Autodesk Fusion 360 part; units mm, degrees
(part 3 of 3)
  spline S37 degree 5 poles (17.7781, 0.5617) (17.7707, 0.5659) (17.756, 0.5742) (17.7338, 0.5867) (17.7042, 0.6032) (17.6672, 0.6236) (17.6301, 0.6437) (17.593, 0.6637) (17.5559, 0.6835) (17.5187, 0.7031) (17.4815, 0.7225) (17.4443, 0.7416) (17.407, 0.7606) (17.3696, 0.7793) (17.3323, 0.7978) (17.2949, 0.8161) (17.2574, 0.8342) (17.22, 0.8521) (17.1824, 0.8698) (17.1449, 0.8872) (17.1073, 0.9045) (17.0697, 0.9215) (17.0321, 0.9382) (16.9944, 0.9548) (16.9567, 0.9711) (16.919, 0.9872) (16.8813, 1.0031) (16.8435, 1.0187) (16.8057, 1.0341) (16.7678, 1.0493) (16.73, 1.0642) (16.6921, 1.0789) (16.6542, 1.0933) (16.6163, 1.1075) (16.5783, 1.1214) (16.5403, 1.1351) (16.5023, 1.1486) (16.4643, 1.1618) (16.4263, 1.1747) (16.3882, 1.1874) (16.3501, 1.1998) (16.312, 1.2119) (16.2739, 1.2238) (16.2358, 1.2354) (16.1976, 1.2467) (16.1595, 1.2577) (16.1213, 1.2684) (16.0831, 1.2789) (16.0449, 1.2891) (16.0067, 1.2989) (15.9685, 1.3085) (15.9303, 1.3177) (15.892, 1.3266) (15.8538, 1.3352) (15.8155, 1.3434) (15.7773, 1.3513) (15.7391, 1.3589) (15.7008, 1.3662) (15.6625, 1.3731) (15.6243, 1.3797) (15.5861, 1.3859) (15.5478, 1.3915) (15.5096, 1.3966) (15.4714, 1.4011) (15.4332, 1.4052) (15.395, 1.4089) (15.3568, 1.4124) (15.3186, 1.4156) (15.2805, 1.4184) (15.2424, 1.4204) (15.2044, 1.4214) (15.174, 1.4209) (15.1513, 1.4197) (15.1361, 1.4185) (15.1285, 1.4178) knots -1 -1 -1 -1 -1 -1 -0.98571429 -0.97142857 -0.95714286 -0.94285714 -0.92857143 -0.91428571 -0.9 -0.88571429 -0.87142857 -0.85714286 -0.84285714 -0.82857143 -0.81428571 -0.8 -0.78571429 -0.77142857 -0.75714286 -0.74285714 -0.72857143 -0.71428571 -0.7 -0.68571429 -0.67142857 -0.65714286 -0.64285714 -0.62857143 -0.61428571 -0.6 -0.58571429 -0.57142857 -0.55714286 -0.54285714 -0.52857143 -0.51428571 -0.5 -0.48571429 -0.47142857 -0.45714286 -0.44285714 -0.42857143 -0.41428571 -0.4 -0.38571429 -0.37142857 -0.35714286 -0.34285714 -0.32857143 -0.31428571 -0.3 -0.28571429 -0.27142857 -0.25714286 -0.24285714 -0.22857143 -0.21428571 -0.2 -0.18571429 -0.17142857 -0.15714286 -0.14285714 -0.12857143 -0.11428571 -0.1 -0.08571429 -0.07142857 -0.05714286 -0.04285714 -0.02857143 -0.01428571 0 0 0 0 0 0
  line L37 (15.1285, 1.4178) -> (14.5093, 1.3603)
  arc A75 (14.0753, 1.7104) -> (14.5093, 1.3603) centre (14.4723, 1.7586) ccw
  arc A76 (14.0753, 1.7104) -> (13.9149, 2.7228) centre (0, 0) ccw
  arc A77 (14.2195, 3.1899) -> (13.9149, 2.7228) centre (14.3075, 2.7996) ccw
  line L38 (14.2195, 3.1899) -> (14.8262, 3.3266)
  spline S38 degree 5 poles (14.8262, 3.3266) (14.8336, 3.3282) (14.8484, 3.3318) (14.8704, 3.3376) (14.8995, 3.3466) (14.9353, 3.3592) (14.9709, 3.373) (15.0063, 3.3874) (15.0416, 3.4023) (15.0769, 3.4173) (15.112, 3.4327) (15.1471, 3.4484) (15.1821, 3.4645) (15.2168, 3.4811) (15.2515, 3.4983) (15.2859, 3.516) (15.3203, 3.5341) (15.3545, 3.5525) (15.3886, 3.5713) (15.4227, 3.5903) (15.4566, 3.6096) (15.4904, 3.6293) (15.5242, 3.6492) (15.5578, 3.6695) (15.5913, 3.6901) (15.6247, 3.711) (15.658, 3.7322) (15.6911, 3.7537) (15.7242, 3.7754) (15.7572, 3.7974) (15.7901, 3.8197) (15.8229, 3.8422) (15.8556, 3.865) (15.8882, 3.8881) (15.9206, 3.9114) (15.953, 3.935) (15.9853, 3.9588) (16.0175, 3.9828) (16.0496, 4.0071) (16.0816, 4.0317) (16.1134, 4.0564) (16.1452, 4.0814) (16.1769, 4.1066) (16.2085, 4.1321) (16.24, 4.1577) (16.2714, 4.1836) (16.3027, 4.2098) (16.3339, 4.2361) (16.365, 4.2626) (16.396, 4.2894) (16.4269, 4.3163) (16.4577, 4.3435) (16.4884, 4.3709) (16.519, 4.3985) (16.5495, 4.4263) (16.5799, 4.4543) (16.6103, 4.4825) (16.6405, 4.5108) (16.6706, 4.5394) (16.7006, 4.5682) (16.7305, 4.5972) (16.7603, 4.6263) (16.79, 4.6557) (16.8196, 4.6853) (16.8492, 4.715) (16.8786, 4.7449) (16.9079, 4.775) (16.9371, 4.8053) (16.9662, 4.8358) (16.9952, 4.8664) (17.0241, 4.8973) (17.0471, 4.9221) (17.0644, 4.9408) (17.0759, 4.9533) (17.0816, 4.9595) knots 0 0 0 0 0 0 0.01428571 0.02857143 0.04285714 0.05714286 0.07142857 0.08571429 0.1 0.11428571 0.12857143 0.14285714 0.15714286 0.17142857 0.18571429 0.2 0.21428571 0.22857143 0.24285714 0.25714286 0.27142857 0.28571429 0.3 0.31428571 0.32857143 0.34285714 0.35714286 0.37142857 0.38571429 0.4 0.41428571 0.42857143 0.44285714 0.45714286 0.47142857 0.48571429 0.5 0.51428571 0.52857143 0.54285714 0.55714286 0.57142857 0.58571429 0.6 0.61428571 0.62857143 0.64285714 0.65714286 0.67142857 0.68571429 0.7 0.71428571 0.72857143 0.74285714 0.75714286 0.77142857 0.78571429 0.8 0.81428571 0.82857143 0.84285714 0.85714286 0.87142857 0.88571429 0.9 0.91428571 0.92857143 0.94285714 0.95714286 0.97142857 0.98571429 1 1 1 1 1 1
  arc A78 (17.0816, 4.9595) -> (16.7344, 6.028) centre (0, 0) ccw
  spline S39 degree 5 poles (16.7344, 6.028) (16.7261, 6.0297) (16.7095, 6.033) (16.6846, 6.038) (16.6513, 6.0445) (16.6098, 6.0525) (16.5683, 6.0602) (16.5269, 6.0678) (16.4854, 6.0751) (16.444, 6.0823) (16.4027, 6.0892) (16.3613, 6.0959) (16.32, 6.1024) (16.2787, 6.1087) (16.2374, 6.1147) (16.1962, 6.1206) (16.155, 6.1262) (16.1138, 6.1317) (16.0727, 6.1369) (16.0316, 6.1419) (15.9906, 6.1466) (15.9495, 6.1512) (15.9086, 6.1555) (15.8676, 6.1596) (15.8267, 6.1635) (15.7859, 6.1672) (15.7451, 6.1706) (15.7043, 6.1738) (15.6636, 6.1767) (15.6229, 6.1795) (15.5823, 6.182) (15.5417, 6.1842) (15.5012, 6.1862) (15.4608, 6.188) (15.4204, 6.1895) (15.38, 6.1908) (15.3397, 6.1919) (15.2995, 6.1927) (15.2593, 6.1932) (15.2192, 6.1935) (15.1791, 6.1935) (15.1392, 6.1933) (15.0992, 6.1928) (15.0594, 6.192) (15.0196, 6.191) (14.9799, 6.1897) (14.9403, 6.1881) (14.9008, 6.1862) (14.8613, 6.1841) (14.8219, 6.1817) (14.7826, 6.179) (14.7434, 6.176) (14.7043, 6.1726) (14.6653, 6.1689) (14.6264, 6.1649) (14.5875, 6.1606) (14.5488, 6.156) (14.5102, 6.1511) (14.4717, 6.1459) (14.4332, 6.1404) (14.395, 6.1344) (14.3569, 6.1279) (14.3189, 6.121) (14.2812, 6.1135) (14.2436, 6.1055) (14.2061, 6.0973) (14.1687, 6.0888) (14.1315, 6.08) (14.0943, 6.0709) (14.0575, 6.0611) (14.021, 6.0502) (13.9923, 6.0404) (13.971, 6.0322) (13.957, 6.0264) (13.95, 6.0234) knots -1 -1 -1 -1 -1 -1 -0.98571429 -0.97142857 -0.95714286 -0.94285714 -0.92857143 -0.91428571 -0.9 -0.88571429 -0.87142857 -0.85714286 -0.84285714 -0.82857143 -0.81428571 -0.8 -0.78571429 -0.77142857 -0.75714286 -0.74285714 -0.72857143 -0.71428571 -0.7 -0.68571429 -0.67142857 -0.65714286 -0.64285714 -0.62857143 -0.61428571 -0.6 -0.58571429 -0.57142857 -0.55714286 -0.54285714 -0.52857143 -0.51428571 -0.5 -0.48571429 -0.47142857 -0.45714286 -0.44285714 -0.42857143 -0.41428571 -0.4 -0.38571429 -0.37142857 -0.35714286 -0.34285714 -0.32857143 -0.31428571 -0.3 -0.28571429 -0.27142857 -0.25714286 -0.24285714 -0.22857143 -0.21428571 -0.2 -0.18571429 -0.17142857 -0.15714286 -0.14285714 -0.12857143 -0.11428571 -0.1 -0.08571429 -0.07142857 -0.05714286 -0.04285714 -0.02857143 -0.01428571 0 0 0 0 0 0
  line L39 (13.95, 6.0234) -> (13.3788, 5.7774)
  arc A79 (12.8578, 5.9762) -> (13.3788, 5.7774) centre (13.2206, 6.1448) ccw
  arc A80 (12.8578, 5.9762) -> (12.3925, 6.8895) centre (0, 0) ccw
  circle A81 centre (0, 0) radius 25
  dimension "d30" = 50
  constraint coincident A0.centre A2.centre
  measures "d30" diameter of A81
extrude "Extrude11" add sketch "Sketch7" along normal blind 5 contours A1 L0 S0 A2 S1 L1 A3 A4 A5 L2 S2 A6 S3 L3 A7 A8 A9 L4 S4 A10 S5 L5 A11 A12 A13 L6 S6 A14 S7 L7 A15 A16 A17 L8 S8 A18 S9 L9 A19 A20 A21 L10 S10 A22 S11 L11 A23 A24 A25 L12 S12 A26 S13 L13 A27 A28 A29 L14 S14 A30 S15 L15 A31 A32 A33 L16 S16 A34 S17 L17 A35 A36 A37 L18 S18 A38 S19 L19 A39 A40 A41 L20 S20 A42 S21 L21 A43 A44 A45 L22 S22 A46 S23 L23 A47 A48 A49 L24 S24 A50 S25 L25 A51 A52 A53 L26 S26 A54 S27 L27 A55 A56 A57 L28 S28 A58 S29 L29 A59 A60 A61 L30 S30 A62 S31 L31 A63 A64 A65 L32 S32 A66 S33 L33 A67 A68 A69 L34 S34 A70 S35 L35 A71 A72 A73 L36 S36 A74 S37 L37 A75 A76 A77 L38 S38 A78 S39 L39 A79 A80 | A81 in component "Spur Gear (20 teeth)"
component "Spur Gear (20 teeth)" placed x (1, 0, 0) y (0, 1, 0) z (0, 0, 1) at (0, 0, 0)
